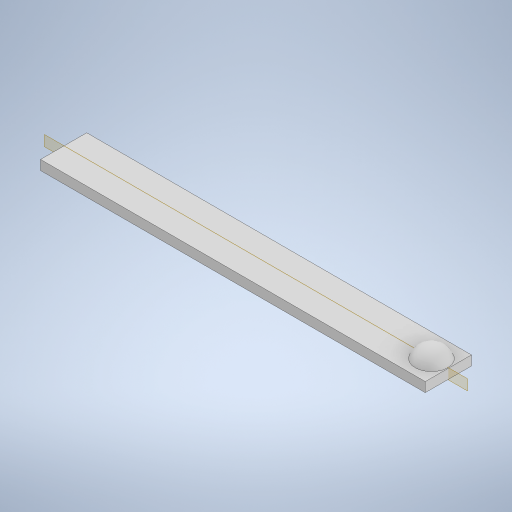
# Autodesk Inventor part: strain sensor silicone
Saved by Autodesk Inventor 2024.2 (Build 282272000, 272)
## iProperties
Created: 2025-02-11
Part Number: strain sensor silicone
Material: Generic
Document SubType Name: Modeling
Designer: Tom
Density: 1 g/cm^3
Appearance: Default
Author: Tom
Autodesk Inventor part; units mm, degrees
ref_plane "YZ Plane" through (0, 0, 0) normal (1, 0, 0) x (0, 1, 0)
ref_plane "XZ Plane" through (0, 0, 0) normal (0, 1, 0) x (-1, 0, 0)
ref_plane "XY Plane" through (0, 0, 0) normal (0, 0, 1) x (1, 0, 0)
sketch "Sketch1" plane through (0, 0, 0) normal (0, 1, 0) x (-1, 0, 0)
  line L0 (0, 0) -> (63.5, 0)
  line L1 (63.5, 0) -> (63.5, -7.62)
  line L2 (63.5, -7.62) -> (0, -7.62)
  line L3 (0, -7.62) -> (0, 0)
  dimension "d0" = 7.62
  dimension "d1" = 63.5
  constraints: 8 end point, 2 parallel, 1 horizontal, 1 perpendicular
  measures "d0" distance of L2.end L0.start
  measures "d1" distance of L1.end L2.end
extrude "Extrusion1" add sketch "Sketch1" along normal blind 1.5875
ref_plane "Work Plane1" through (-63.5, 0, -3.81) normal (0, 0, 1) x (1, 0, 0)
sketch "Sketch2" plane through (-63.5, 0, -3.81) normal (0, 0, 1) x (1, 0, 0)
  arc A0 (63.3849, 1.5875) -> (60.7062, 3.5875) centre (60.7062, 0.7937) ccw
  line L0 (63.5, 1.5875) -> (0, 1.5875) projected
  line L1 (63.5, 1.5875) -> (60.7062, 1.5875)
  line L2 (60.7062, 3.5875) -> (60.7062, 1.5875)
  line L3 (60.7062, 1.5875) -> (60.7062, 0.676)
  point P0 (63.5, 0)
  constraints: 6 end point, 2 point on circle, 2 vertical, 1 centre point, 1 point on line
revolve "Revolution1" add sketch "Sketch2" angle 360 about axis through (-2.7938, 3.5875, -3.81) along (0, -1, 0)
body "Solid1"
